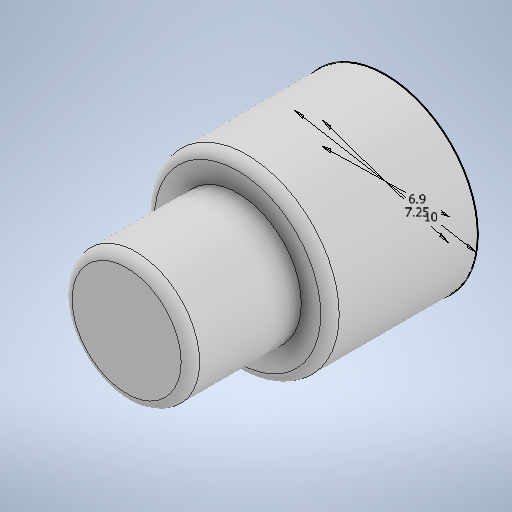
# Autodesk Inventor part: button
Saved by Autodesk Inventor 2025 (Build 290162010, 162A)
## iProperties
Created: 2025-11-21
Part Number: button
Material: Generic
Document SubType Name: Modeling
Designer: vaugerbird
Density: 1 g/cm^3
Appearance: Default
Author: vaugerbird
Autodesk Inventor part; units mm, degrees
ref_plane "YZ Plane" through (0, 0, 0) normal (1, 0, 0) x (0, 1, 0)
ref_plane "XZ Plane" through (0, 0, 0) normal (0, 1, 0) x (-1, 0, 0)
ref_plane "XY Plane" through (0, 0, 0) normal (0, 0, 1) x (1, 0, 0)
sketch "Sketch1" plane through (0, 0, 0) normal (0, 0, 1) x (1, 0, 0)
  circle A0 centre (0, 0) radius 5
  circle A1 centre (0, 0) radius 3.45
  circle A2 centre (0, 0) radius 3.625
  dimension "d0" = 10
  dimension "d1" = 6.9
  dimension "d2" = 7.25
  constraints: 3 centre point, 3 coincident
  measures "d0" diameter of A0
  measures "d1" diameter of A1
  measures "d2" diameter of A2
extrude "Extrusion1" add sketch "Sketch1" along normal blind 8 contours A0 | A1 | A2
extrude "Extrusion2" add sketch "Sketch1" along normal blind 14 contours A1
extrude "Extrusion3" cut sketch "Sketch1" along normal blind 4 contours A1 | A2
draft "FaceDraft1" angle 2.5 pull direction (0, 0, -1) faces at (3.6132, -0.2917, 2.6667) fixed edges at (-3.625, 0, 4)
fillet "Fillet1" radius 0.5 3 edges at (-3.45, 0, 14) (-5, 0, 8) (-3.7996, 0, 0)
body "Solid1"
